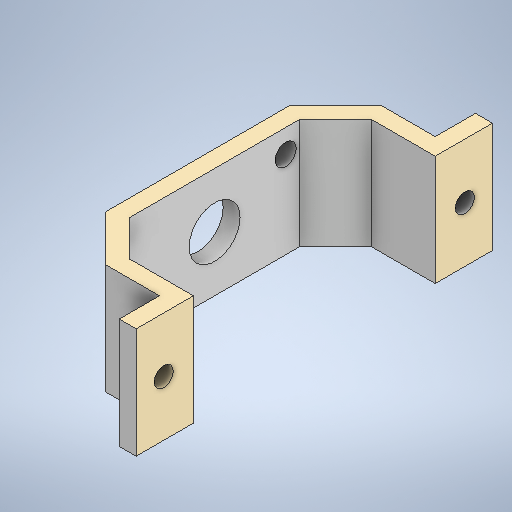
# Autodesk Inventor part: Pulley Bearing Support.-3
Saved by Autodesk Inventor 2025 (Build 290162000, 162)
## iProperties
Created: 2025-07-19
Part Number: Pulley Bearing Support.-3
Material: Generic
Document SubType Name: Modeling
Designer: yshis
Density: 1 g/cm^3
Appearance: Default
Author: yshis
Autodesk Inventor part; units mm, degrees
ref_plane "YZ Plane" through (0, 0, 0) normal (1, 0, 0) x (0, 1, 0)
ref_plane "XZ Plane" through (0, 0, 0) normal (0, 1, 0) x (-1, 0, 0)
ref_plane "XY Plane" through (0, 0, 0) normal (0, 0, 1) x (1, 0, 0)
sketch "Sketch1" plane through (0, 0, 0) normal (0, 1, 0) x (-1, 0, 0)
  line L0 (0.1637, 10.9307) -> (0.1637, -2.5693)
  line L1 (0.1637, -59.5693) -> (0.1637, -73.0693)
  line L2 (0.1637, -2.5693) -> (15.1637, -2.5693)
  line L3 (0.1637, -59.5693) -> (15.1637, -59.5693)
  line L4 (15.1637, -2.5693) -> (23.6637, -11.0693)
  line L5 (15.1637, -59.5693) -> (23.6637, -51.0693)
  line L6 (23.6637, -11.0693) -> (23.6637, -51.0693)
  line L7 (4.1637, -73.0693) -> (4.1637, -63.5693)
  line L8 (4.1637, -63.5693) -> (16.8205, -63.5693)
  line L9 (16.8205, -63.5693) -> (27.6637, -52.7262)
  line L10 (27.6637, -52.7262) -> (27.6637, -9.4125)
  line L11 (27.6637, -9.4125) -> (16.8205, 1.4307)
  line L12 (16.8205, 1.4307) -> (4.1637, 1.4307)
  line L13 (4.1637, 1.4307) -> (4.1637, 10.9307)
  line L14 (4.1637, 10.9307) -> (0.1637, 10.9307)
  line L15 (4.1637, -73.0693) -> (0.1637, -73.0693)
  point P0 (0, 0)
  point P1 (0.1637, 4.1807)
  dimension "d5" = 13.5
  dimension "d6" = 13.5
  dimension "d98" = 0
  dimension "d100" = 15
  dimension "d101" = 15
  dimension "d103" = 135
  dimension "d104" = 135
  dimension "d106" = 23.5
  dimension "d107" = 4
  dimension "d111" = 84
  constraints: 32 end point, 3 horizontal, 3 vertical, 1 midpoint, 1 parallel, 6 other
  measures "d5" distance of L1.start L1.end
  measures "d6" distance of L0.start L0.end
  measures "d98" distance from line of L1 point (0.164, 4.181)
  measures "d100" distance of L0.end L2.end
  measures "d101" distance of L1.start L3.end
  measures "d103" angle of L4 L2
  measures "d104" angle of L3 L5
  measures "d106" distance from line of L6 L0.end
  measures "d107" distance between parallel lines of L6 L10
  measures "d111" distance of L0.start L1.end
extrude "Extrusion1" add sketch "Sketch1" along normal blind 26
sketch "Sketch2" plane through (-0.1637, 0, 10.9307) normal (1, 0, 0) x (0, 0, -1)
  circle A0 centre (6.5, 13) radius 2.25
  line L0 (0, 0) -> (0, 26) projected
  line L1 (0, 0) -> (13.5, 0) projected
  circle A1 centre (77.5, 13) radius 2.25
  point P0 (10.9307, 0)
  dimension "d23" = 4.5
  dimension "d29" = 6.5
  dimension "d30" = 13
  dimension "d93" = 71
  constraints: 2 centre point, 1 horizontal, 2 other
  measures "d23" diameter of A0
  measures "d29" distance from line of L0 A0.centre
  measures "d30" distance from line of A0.centre L1
  measures "d93" distance of A0.centre A1.centre
extrude "Extrusion2" cut sketch "Sketch2" against normal blind 10
sketch "Sketch7" plane through (-27.6637, 0, -52.7262) normal (-1, 0, 0) x (0, 0, 1)
  circle A0 centre (21.6569, 13) radius 6
  line L0 (63.6569, 0) -> (63.6569, 26) projected
  line L1 (0, 0) -> (43.3137, 0) projected
  point P0 (52.7262, 0)
  point P1 (21.6569, 0)
  dimension "d108" = 12
  dimension "d109" = 42
  dimension "d110" = 13
  constraints: 1 centre point, 1 midpoint
  measures "d108" diameter of A0
  measures "d109" distance from line of A0.centre L0
  measures "d110" distance of point (21.657, 0) A0.centre
extrude "Extrusion7" cut sketch "Sketch7" against normal blind 10
sketch "Sketch8" plane through (-27.6637, 0, -52.7262) normal (-1, 0, 0) x (0, 0, 1)
  circle A0 centre (21.6569, 13) radius 6 projected
  circle A1 centre (21.6569, 13) radius 18.35
  circle A2 centre (38.4042, 5.5) radius 2.5
  line L0 (0, 0) -> (43.3137, 0) projected
  circle A3 centre (4.9095, 20.5) radius 2.5
  point P0 (52.7262, 0)
  dimension "d114" = 36.7
  dimension "d115" = 5
  dimension "d116" = 5.5
  dimension "d119" = 360
  constraints: 3 coincident, 2 centre point, 8 other
  measures "d115" diameter of A2
  measures "d116" distance from line of L0 A2.centre
extrude "Extrusion8" cut sketch "Sketch8" against normal blind 10 contours A3 A1 | A1 A3 | A2 A1 | A1 A2
sketch "Sketch9" plane through (-4.1637, 0, 1.4307) normal (-1, 0, 0) x (0, 0, 1)
  circle A0 centre (3, 13.0738) radius 4
  circle A1 centre (-68, 13.0738) radius 4
  point P0 (-1.4307, 0)
  dimension "d123" = 8
  dimension "d124" = 8
  constraints: 2 centre point
  measures "d123" diameter of A0
  measures "d124" diameter of A1
extrude "Extrusion9" cut sketch "Sketch9" along normal blind 4
equation "\"d5\" = d6"
equation "\"d29\" = -0.5 * d33 + 0.5 * d17"
equation "\"d30\" = 0.5 * d20"
equation "\"d33\" = 71"
equation "\"d17\" = 84"
equation "\"d20\" = 26"
body "Solid1"
